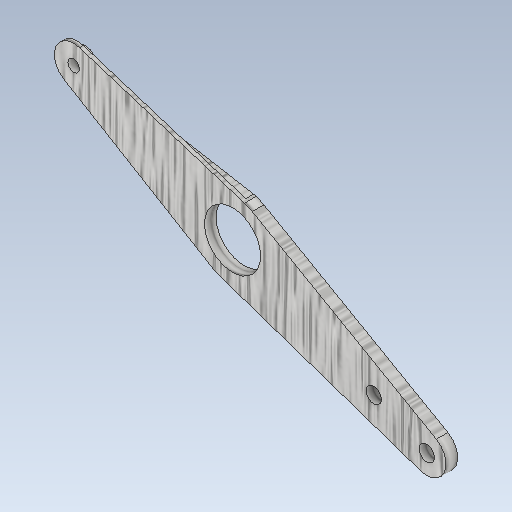
# Autodesk Inventor part: アーム中間節
Saved by Autodesk Inventor 2020 (Build 240168000, 168)
## iProperties
Created: 2019-12-03
Part Number: アーム中間節
Material: アルミニウム 7075
Document SubType Name: Modeling
Designer: tanjihayato
Density: 2.81 g/cm^3
Appearance: サテン - ブラシ仕上げ 重厚
Mass: 8.5012 g
Surface Area: 39.9096 cm^2
Volume: 3.02534 cm^3
Author: tanjihayato
Autodesk Inventor part; units mm, degrees
note: some values were not read from the file. Chosen so that the rebuilt part matches the saved one: sketch regions of "押し出し1"; sketch regions of "押し出し2".
ref_plane "YZ Plane" through (0, 0, 0) normal (1, 0, 0) x (0, 1, 0)
ref_plane "XZ Plane" through (0, 0, 0) normal (0, 1, 0) x (-1, 0, 0)
ref_plane "XY Plane" through (0, 0, 0) normal (0, 0, 1) x (1, 0, 0)
sketch "スケッチ1" plane through (0, 0, 0) normal (0, 0, 1) x (1, 0, 0)
  line L0 (-170.6512, -31.4118) -> (202.8656, -31.4118) construction
  circle A0 centre (-14, -17.4118) radius 14 construction
  circle A1 centre (14, -17.4118) radius 14 construction
  circle A2 centre (-28.0204, 0.0121) radius 20.05 construction
  circle A3 centre (-28.0204, 0.0121) radius 5.05 construction
  circle A4 centre (8.8763, 3.8907) radius 32.05 construction
  circle A5 centre (8.8763, 3.8907) radius 10.1 construction
  circle A6 centre (54.047, 13.5882) radius 36.1 construction
  line L1 (-170.915, -81.4118) -> (490.0044, -81.4118)
  circle A7 centre (-28.0204, 0.0121) radius 22.342 construction
  circle A8 centre (-39.4931, 19.1835) radius 14 construction
  circle A9 centre (-49.0547, 7.5438) radius 14 construction
  circle A10 centre (-49.0547, -7.5196) radius 14 construction
  circle A11 centre (-39.4931, -19.1593) radius 14 construction
  circle A12 centre (8.8763, 3.8907) radius 33.05 construction
  circle A13 centre (54.047, 13.5882) radius 38.1 construction
  line L2 (-11.5565, -29.1593) -> (4.2969, -29.1593) construction
  line L3 (-67.2952, 44.8622) -> (-67.2952, -57.3934) construction
  line L4 (-149.4523, -1.6098) -> (-132.6633, -31.6026)
  line L5 (-132.7701, -31.4118) -> (-132.7701, 74.0456)
  circle A14 centre (-11.4931, -19.1593) radius 14 construction
  line L6 (-197.2268, -33.1593) -> (179.6604, -33.1593) construction
  circle A15 centre (54.047, 13.5882) radius 4.025 construction
  circle A16 centre (54.047, 13.5882) radius 6 construction
  circle A17 centre (-39.4931, 19.1835) radius 5
  circle A18 centre (-49.0547, 7.5438) radius 5
  circle A19 centre (-49.0547, -7.5196) radius 5
  circle A20 centre (-39.4931, -19.1593) radius 5
  circle A21 centre (-39.4931, 19.1835) radius 8 construction
  circle A22 centre (-49.0547, 7.5438) radius 8 construction
  circle A23 centre (-49.0547, -7.5196) radius 8 construction
  circle A24 centre (-39.4931, -19.1593) radius 8 construction
  circle A25 centre (-28.0204, 0.0121) radius 4.5
  circle A26 centre (8.8763, 3.8907) radius 7.5
  line L7 (-17.5497, 32.3149) -> (-46.3578, 15.0755) construction
  line L8 (-46.3578, 15.0755) -> (-51.7515, 0.0121) construction
  line L9 (-51.7515, 0.0121) -> (-46.3578, -15.0513) construction
  line L10 (-46.3578, -15.0513) -> (-37.9391, -20.0892) construction
  circle A27 centre (-32.6283, 23.2915) radius 1.3
  circle A28 centre (-46.3578, 15.0755) radius 1.3
  circle A29 centre (-51.7515, 0.0121) radius 1.3
  circle A30 centre (-46.3578, -15.0513) radius 1.3
  circle A31 centre (-32.6283, -23.2673) radius 1.3
  line L11 (-67.2952, 23.1796) -> (-67.2952, -18.1327)
  arc A32 (79.2003, -37.212) -> (87.3507, -31.2711) centre (80.4159, -30.3183) ccw
  arc A33 (8.1864, 50.8943) -> (0.9804, 51.9708) centre (3.7003, 45.5208) ccw
  line L12 (-52.2685, -33.1593) -> (56.2168, -33.1593)
  line L13 (56.2168, -33.1593) -> (79.2003, -37.212)
  arc A34 (92.7831, 8.2659) -> (29.742, 44.2162) centre (54.047, 13.5882) ccw
  line L14 (87.3507, -31.2711) -> (92.7831, 8.2659)
  line L15 (0.9804, 51.9708) -> (-67.2952, 23.1796)
  circle A35 centre (34.0114, -24.0061) radius 4.5 construction
  circle A36 centre (34.0114, -24.0061) radius 1.5
  circle A37 centre (-21.4477, 26.0369) radius 4.5 construction
  circle A38 centre (-21.4477, 26.0369) radius 1.5
  circle A39 centre (-56.0504, 23.0377) radius 1.5
  circle A40 centre (-56.0504, 23.0377) radius 3 construction
  circle A41 centre (-56.0504, 23.0377) radius 4.5 construction
  circle A42 centre (-64.2952, 0.0121) radius 1.5
  circle A43 centre (-64.2952, 0.0121) radius 3 construction
  circle A44 centre (-64.2952, 0.0121) radius 4.3311 construction
  line L16 (54.047, 13.5882) -> (99.37, -7.5264)
  line L17 (99.37, -7.5264) -> (58.3399, 10.9541)
  line L18 (58.3399, 10.9541) -> (30.7326, 32.4678)
  line L19 (30.7326, 32.4678) -> (54.047, 13.5882)
  line L20 (99.37, -7.5264) -> (491.4359, -184.1173)
  line L21 (-183.2789, 162.2213) -> (-183.2789, -125.2315)
  line L22 (516.7211, 155.5913) -> (516.7211, -155.5644)
  circle A45 centre (99.37, -7.5264) radius 7.25
  line L23 (149.518, -30.1136) -> (397.5027, -198.9436) construction
  line L24 (220.2014, -78.2354) -> (225.3858, -8.4277) construction
  circle A46 centre (3.7003, 45.5208) radius 4
  circle A47 centre (135.8413, -23.9534) radius 2
  circle A48 centre (149.518, -30.1136) radius 2
  arc A49 (147.9092, -34.8477) -> (151.9972, -25.7715) centre (149.518, -30.1136) ccw
  line L25 (147.9092, -34.8477) -> (96.0719, -17.2312)
  line L26 (151.9972, -25.7715) -> (104.4523, 1.3749)
  circle A50 centre (30.7326, 32.4678) radius 2
  circle A51 centre (-16.1798, -24.0771) radius 4.5 construction
  circle A52 centre (-16.1798, -24.0771) radius 1.5
  line L27 (-67.2952, -18.1327) -> (-52.2685, -33.1593)
  circle A53 centre (-56.0504, -23.0135) radius 1.5
  circle A54 centre (-56.0504, -23.0135) radius 3 construction
  circle A55 centre (30.7326, 32.4678) radius 4
  arc A56 (56.8403, 15.6972) -> (51.3644, 11.3402) centre (54.047, 13.5882) ccw construction
  line L28 (96.4916, -6.1854) -> (101.9705, -5.7041) construction
  line L29 (101.9705, -5.7041) -> (99.6479, -10.6896) construction
  line L30 (99.6479, -10.6896) -> (96.4916, -6.1854) construction
  circle A57 centre (99.6479, -10.6896) radius 1.5
  circle A58 centre (101.9705, -5.7041) radius 1.5
  circle A59 centre (96.4916, -6.1854) radius 1.5
  circle A60 centre (99.37, -7.5264) radius 6
  arc A61 (97.7876, -15.8778) -> (97.5111, 0.7679) centre (99.37, -7.5264) ccw
  arc A62 (56.8403, 15.6972) -> (97.5111, 0.7679) centre (88.7632, 39.7996) ccw
  arc A63 (51.3644, 11.3402) -> (97.7876, -15.8778) centre (112.6811, 62.7237) ccw
  circle A64 centre (54.047, 13.5882) radius 8.5 construction
  line L31 (102.9595, 0.1786) -> (57.6365, 21.2931) construction
  line L32 (50.4575, 5.8833) -> (95.7806, -15.2313) construction
  circle A65 centre (12.7384, 41.2415) radius 3 construction
  circle A66 centre (12.7384, 41.2415) radius 4.5 construction
  circle A67 centre (12.7384, 41.2415) radius 1.5
  circle A68 centre (80.4159, -30.3183) radius 4
  circle A69 centre (69.7531, -26.0108) radius 1.5
  circle A70 centre (69.7531, -26.0108) radius 4.5 construction
  circle A71 centre (-56.0504, -23.0135) radius 4.5 construction
  line L33 (8.1864, 50.8943) -> (15.9809, 44.3871)
  arc A72 (15.9809, 44.3871) -> (29.742, 44.2162) centre (22.9664, 52.7545) ccw
  circle A73 centre (-5.4761, 38.5895) radius 1.5
  circle A74 centre (-5.4761, 38.5895) radius 4.5 construction
  circle A75 centre (54.047, 13.5882) radius 50 construction
  circle A76 centre (3.7003, 45.5208) radius 2
  circle A77 centre (80.4159, -30.3183) radius 2
  circle A78 centre (54.047, 13.5882) radius 1.5
  circle A79 centre (58.3399, 10.9541) radius 1.5
  circle A80 centre (58.3399, 10.9541) radius 3
  arc A81 (59.8474, 15.7214) -> (55.7687, 6.6659) centre (58.3399, 10.9541) ccw
  line L34 (94.099, -16.3172) -> (55.7687, 6.6659)
  line L35 (59.8474, 15.7214) -> (102.4604, 2.2467)
  arc A82 (104.4523, 1.3749) -> (102.4604, 2.2467) centre (99.37, -7.5264) ccw
  arc A83 (94.099, -16.3172) -> (96.0719, -17.2312) centre (99.37, -7.5264) ccw
  circle A84 centre (30.7326, 32.4678) radius 5.025
  circle A85 centre (30.7326, 32.4678) radius 8.025
  circle A86 centre (58.3399, 10.9541) radius 4.025
  circle A87 centre (58.3399, 10.9541) radius 7.025
  line L36 (25.9827, 25.9995) -> (54.1819, 5.2918)
  line L37 (53.3095, 15.8577) -> (37.1861, 27.6978)
  line L38 (65.3516, 11.3852) -> (66.2721, -3.5865)
  line L39 (66.2721, -3.5865) -> (54.1819, 5.2918)
  line L40 (66.4799, 8.6117) -> (69.0337, -1.2879)
  line L41 (66.4799, 8.6117) -> (101.8062, 2.4535)
  point P0 (0, 0)
  point P1 (0, 0)
  point P2 (-49.0547, 7.5438)
  point P3 (-49.0547, -7.5196)
  dimension "d88" = 100
  dimension "d0" = 40.1
  dimension "d1" = 10.1
  dimension "d2" = 64.1
  dimension "d3" = 20.2
  dimension "d4" = 72.2
  dimension "d5" = 95
  dimension "d6" = 44.684
  dimension "d7" = 28
  dimension "d8" = 28
  dimension "d9" = 28
  dimension "d10" = 28
  dimension "d11" = 1
  dimension "d12" = 2
  dimension "d13" = 4
  dimension "d14" = 8.05
  dimension "d15" = 12
  dimension "d16" = 10
  dimension "d17" = 10
  dimension "d18" = 10
  dimension "d19" = 10
  dimension "d20" = 3
  dimension "d21" = 3
  dimension "d22" = 3
  dimension "d23" = 3
  dimension "d24" = 9
  dimension "d25" = 15
  dimension "d26" = 2.6
  dimension "d27" = 2.6
  dimension "d28" = 2.6
  dimension "d29" = 2.6
  dimension "d30" = 2.6
  dimension "d31" = 1
  dimension "d32" = 9
  dimension "d33" = 3
  dimension "d34" = 9
  dimension "d35" = 3
  dimension "d36" = 3
  dimension "d37" = 6
  dimension "d38" = 9
  dimension "d39" = 3
  dimension "d40" = 6
  dimension "d41" = 50
  dimension "d42" = 45
  dimension "d43" = 35
  dimension "d44" = 30
  dimension "d45" = 39
  dimension "d46" = 430
  dimension "d47" = 700
  dimension "d48" = 14.5
  dimension "d49" = 300
  dimension "d50" = 10
  dimension "d51" = 70
  dimension "d52" = 120
  dimension "d53" = 140
  dimension "d54" = 8
  dimension "d55" = 4
  dimension "d56" = 4
  dimension "d57" = 15
  dimension "d58" = 40
  dimension "d59" = 10
  dimension "d60" = 4
  dimension "d61" = 9
  dimension "d62" = 3
  dimension "d63" = 3
  constraints: 84 centre point, 84 end point, 60 tangent, 47 coincident, 39 point on circle, 15 point on line, 4 midpoint, 4 vertical, 2 collinear, 2 horizontal, 1 parallel, 1 vertical alignment, 23 other
  measures "d0" diameter of A2
  measures "d1" diameter of A3
  measures "d2" diameter of A4
  measures "d3" diameter of A5
  measures "d4" diameter of A6
  measures "d5" distance from line of L1 A6.centre
  measures "d6" diameter of A7
  measures "d7" diameter of A8
  measures "d8" diameter of A9
  measures "d9" diameter of A10
  measures "d10" diameter of A11
  measures "d11" radial gap between concentric circles of A4 A12
  measures "d12" radial gap between concentric circles of A6 A13
  measures "d13" distance between parallel lines of L6 L2
  measures "d14" diameter of A15
  measures "d15" diameter of A16
  measures "d16" diameter of A17
  measures "d17" diameter of A18
  measures "d18" diameter of A19
  measures "d19" diameter of A20
  measures "d20" radial gap between concentric circles of A17 A21
  measures "d24" diameter of A25
  measures "d25" diameter of A26
  measures "d26" diameter of A27
  measures "d27" diameter of A28
  measures "d28" diameter of A29
  measures "d29" diameter of A30
  measures "d30" diameter of A31
  measures "d31" radial gap between concentric circles of A13 A34
  measures "d32" diameter of A35
  measures "d33" diameter of A36
  measures "d34" diameter of A37
  measures "d35" diameter of A38
  measures "d36" diameter of A39
  measures "d37" diameter of A40
  measures "d38" diameter of A41
  measures "d39" diameter of A42
  measures "d40" diameter of A43
  measures "d41" distance of L16.start L16.end
  measures "d42" distance of L16.end L17.end
  measures "d43" distance of L17.end L18.end
  measures "d44" distance of L18.end L16.start
  measures "d45" angle of L0 L19
  measures "d46" distance of L16.end L20.end
  measures "d47" distance between parallel lines of L22 L21
  measures "d48" diameter of A45
  measures "d49" distance of L23.start L23.end
  measures "d50" angle of L20 L23
  measures "d51" distance of L24.start L24.end
  measures "d52" angle of L23 L24
  measures "d53" distance of L16.end L24.start
  measures "d54" diameter of A46
  measures "d55" diameter of A47
  measures "d56" diameter of A48
  measures "d57" distance of L23.start A47.centre
  measures "d58" distance of A47.centre A45.centre
  measures "d59" diameter of A49
  measures "d60" diameter of A50
  measures "d61" diameter of A51
  measures "d62" diameter of A52
  measures "d63" diameter of A53
extrude "押し出し1" add sketch "スケッチ1" along normal blind 3 contours L35 L41 L14 | L14 L41 L40 L16 L38 A87 L35 | L34 L40 A62 L17 L14 | L14 L17 A45 L20 A61 A63 L34 | A63 A61 L20 A47 A48 A49 L25 A83 L34 | L41 L35 A82 L26 A49 L20 A48 A47 A61 A62 L14 | L14 A62 L16 L40 L41 | A87 L16 A62 A86 A78 A81 L35 | L17 A62 L16 L14 | L14 L16 A45 L17 | L34 L38 A62 L40 | L34 A87 A62 L38 | A62 A61 L20 A45 L16 L14 | L14 L16 A62 | L38 L16 A87 | A62 L40 L17 | L17 L40 L16 A62 | A62 L38 L17 L40 | A81 A63 | A63 A81 A78 A86 L17 A62 A87 L34 | A62 A87 L17 L38 | L40 L17 L38 L16 | A78 A86 L18 A81 | L38 L17 A87 L16 | A62 L17 A87 | A86 A62 A80 L18 A78 | A78 L18 A86 | L18 A86 L16 A81 | A87 L17 A62 L16 | A81 L16 A86 A78 | L17 A86 L16 A62 | A86 A62 A80 | L18 A78 L16 A86 | L16 A86 A62 | A86 L16 A78 | A78 L16 A80 L17 A86 | L17 A80 L16 A86 | L18 A80 L16 A78 | A80 A62 | A62 A80 L16 A79 L18 | L16 A80 A62 A86 | A80 L16 L18 A79 L17 | L17 A79 L16 A80 | L18 L16 A80 | L16 A79 L18
extrude "押し出し2" cut sketch "スケッチ1" along normal blind 2 contours L35 L41 L14 | L14 L41 L40 L16 L38 A87 L35 | A87 L16 A62 A86 A78 A81 L35 | L34 L38 A62 L40 | L34 A87 A62 L38 | L38 L16 A87 | A62 L38 L17 L40 | A81 A63 | A63 A81 A78 A86 L17 A62 A87 L34 | A62 A87 L17 L38 | L40 L17 L38 L16 | A78 A86 L18 A81 | L38 L17 A87 L16 | A62 L17 A87 | A86 A62 A80 L18 A78 | A78 L18 A86 | L18 A86 L16 A81 | A87 L17 A62 L16 | A81 L16 A86 A78 | L17 A86 L16 A62 | A86 A62 A80 | L18 A78 L16 A86 | L16 A86 A62 | A86 L16 A78 | A78 L16 A80 L17 A86 | L17 A80 L16 A86 | L18 A80 L16 A78 | L16 A80 A62 A86
sketch "スケッチ3" plane through (0, 0, 0) normal (0, 0, -1) x (-1, 0, 0)
  line L0 (-66.4799, 8.6117) -> (-101.8062, 2.4535) projected
  line L1 (-102.4604, 2.2467) -> (-101.8062, 2.4535) projected
  arc A0 (-102.4604, 2.2467) -> (-104.4523, 1.3749) centre (-99.37, -7.5264) ccw projected
  line L2 (-151.9972, -25.7715) -> (-104.4523, 1.3749) projected
  arc A1 (-151.9972, -25.7715) -> (-147.9092, -34.8477) centre (-149.518, -30.1136) ccw projected
  line L3 (-96.0719, -17.2312) -> (-147.9092, -34.8477) projected
  arc A2 (-96.0719, -17.2312) -> (-94.099, -16.3172) centre (-99.37, -7.5264) ccw projected
  line L4 (-69.0337, -1.2879) -> (-94.099, -16.3172) projected
  line L5 (-69.0337, -1.2879) -> (-66.4799, 8.6117) projected
  circle A3 centre (-135.8413, -23.9534) radius 2 projected
  circle A4 centre (-149.518, -30.1136) radius 2 projected
  circle A5 centre (-99.37, -7.5264) radius 7.25 projected
  arc A6 (-101.5559, -0.6137) -> (-102.9648, -1.2303) centre (-99.37, -7.5264) ccw
  line L6 (-101.5559, -0.6137) -> (-101.0932, -0.4674)
  line L7 (-101.0932, -0.4674) -> (-70.5466, 4.8575)
  line L8 (-70.5466, 4.8575) -> (-71.6313, 0.6525)
  line L9 (-71.6313, 0.6525) -> (-95.6417, -13.7443)
  arc A7 (-97.0372, -14.3908) -> (-95.6417, -13.7443) centre (-99.37, -7.5264) ccw
  line L10 (-97.0372, -14.3908) -> (-148.8745, -32.0072)
  arc A8 (-150.5097, -28.3767) -> (-148.8745, -32.0072) centre (-149.518, -30.1136) ccw
  line L11 (-150.5097, -28.3767) -> (-102.9648, -1.2303)
  arc A9 (-131.2941, -26.0327) -> (-134.3851, -19.1702) centre (-135.8413, -23.9534) ccw
  arc A10 (-109.2571, -4.823) -> (-103.8976, -16.7222) centre (-99.37, -7.5264) ccw
  arc A11 (-89.4275, -10.0182) -> (-93.477, 0.8602) centre (-99.37, -7.5264) ccw
  point P0 (0, 0)
  dimension "d111" = 3
  dimension "d113" = 3
  dimension "d114" = 3
  dimension "d115" = 3
  constraints: 12 end point, 12 point on circle, 6 centre point, 6 point on line, 8 other
  measures "d111" distance between parallel lines of L2 L11
  measures "d113" radial gap between concentric circles of A3 A9
  measures "d114" radial gap between concentric circles of A10 A5
  measures "d115" radial gap between concentric circles of A11 A5
extrude "押し出し3" cut sketch "スケッチ3" against normal blind 2 contours L11 A10 L10 A9 | A11 L7 L8 L9
fillet "フィレット1" radius 2 8 edges at (134.3851, -19.1702, 1) (131.2941, -26.0327, 1) (103.8976, -16.7222, 1) (109.2571, -4.823, 1) (93.477, 0.8602, 1) (89.4275, -10.0182, 1) (71.6313, 0.6525, 1) (70.5466, 4.8575, 1)
sketch "スケッチ4" plane through (0, 0, 0) normal (0, 0, -1) x (-1, 0, 0)
  arc A0 (-89.1684, -6.5314) -> (-91.0011, -1.6084) centre (-99.37, -7.5264) ccw projected
  arc A1 (-89.7115, 1.5167) -> (-91.0011, -1.6084) centre (-89.3681, -0.4536) ccw projected
  line L0 (-89.7115, 1.5167) -> (-73.6012, 4.325) projected
  arc A2 (-71.3211, 1.8552) -> (-73.6012, 4.325) centre (-73.2577, 2.3548) ccw projected
  line L1 (-71.3211, 1.8552) -> (-71.4265, 1.4465) projected
  arc A3 (-72.3346, 0.2308) -> (-71.4265, 1.4465) centre (-73.3631, 1.9461) ccw projected
  line L2 (-72.3346, 0.2308) -> (-86.1494, -8.0526) projected
  arc A4 (-89.1684, -6.5314) -> (-86.1494, -8.0526) centre (-87.1779, -6.3373) ccw projected
  arc A5 (-130.8782, -23.3469) -> (-132.0981, -20.6385) centre (-135.8413, -23.9534) ccw projected
  arc A6 (-131.5925, -17.5757) -> (-132.0981, -20.6385) centre (-130.6008, -19.3125) ccw projected
  line L3 (-131.5925, -17.5757) -> (-112.5765, -6.7182) projected
  arc A7 (-109.5905, -8.3034) -> (-112.5765, -6.7182) centre (-111.5848, -8.4551) ccw projected
  arc A8 (-109.5905, -8.3034) -> (-106.725, -14.6655) centre (-99.37, -7.5264) ccw projected
  arc A9 (-107.5166, -17.9521) -> (-106.725, -14.6655) centre (-108.1601, -16.0585) ccw projected
  line L4 (-107.5166, -17.9521) -> (-128.2494, -24.998) projected
  arc A10 (-130.8782, -23.3469) -> (-128.2494, -24.998) centre (-128.893, -23.1043) ccw projected
  line L5 (-66.4799, 8.6117) -> (-101.8062, 2.4535) projected
  line L6 (-102.4604, 2.2467) -> (-101.8062, 2.4535) projected
  arc A11 (-102.4604, 2.2467) -> (-104.4523, 1.3749) centre (-99.37, -7.5264) ccw projected
  line L7 (-151.9972, -25.7715) -> (-104.4523, 1.3749) projected
  arc A12 (-151.9972, -25.7715) -> (-147.9092, -34.8477) centre (-149.518, -30.1136) ccw projected
  line L8 (-96.0719, -17.2312) -> (-147.9092, -34.8477) projected
  arc A13 (-96.0719, -17.2312) -> (-94.099, -16.3172) centre (-99.37, -7.5264) ccw projected
  line L9 (-69.0337, -1.2879) -> (-94.099, -16.3172) projected
  line L10 (-69.0337, -1.2879) -> (-66.4799, 8.6117) projected
  circle A14 centre (-135.8413, -23.9534) radius 2 projected
  circle A15 centre (-149.518, -30.1136) radius 2 projected
  circle A16 centre (-99.37, -7.5264) radius 7.25 projected
  arc A17 (-55.7687, 6.6659) -> (-59.8474, 15.7214) centre (-58.3399, 10.9541) ccw projected
  line L11 (-101.8062, 2.4535) -> (-59.8474, 15.7214) projected
  line L12 (-66.4799, 8.6117) -> (-101.8062, 2.4535) projected
  line L13 (-69.0337, -1.2879) -> (-66.4799, 8.6117) projected
  line L14 (-55.7687, 6.6659) -> (-69.0337, -1.2879) projected
  circle A18 centre (-58.3399, 10.9541) radius 3 projected
  arc A19 (-151.9972, -25.7715) -> (-147.9092, -34.8477) centre (-149.518, -30.1136) ccw projected
  line L15 (-151.9972, -25.7715) -> (-104.4523, 1.3749) projected
  arc A20 (-102.4604, 2.2467) -> (-104.4523, 1.3749) centre (-99.37, -7.5264) ccw projected
  line L16 (-102.4604, 2.2467) -> (-59.8474, 15.7214) projected
  arc A21 (-55.7687, 6.6659) -> (-59.8474, 15.7214) centre (-58.3399, 10.9541) ccw projected
  line L17 (-55.7687, 6.6659) -> (-94.099, -16.3172) projected
  arc A22 (-96.0719, -17.2312) -> (-94.099, -16.3172) centre (-99.37, -7.5264) ccw projected
  line L18 (-96.0719, -17.2312) -> (-147.9092, -34.8477) projected
  circle A23 centre (-135.8413, -23.9534) radius 2 projected
  circle A24 centre (-149.518, -30.1136) radius 2 projected
  circle A25 centre (-99.37, -7.5264) radius 7.25 projected
  circle A26 centre (-58.3399, 10.9541) radius 1.5 projected
  arc A27 (-102.2781, 4.4966) -> (-101.8062, 2.4535) centre (-101.9865, 3.4879) ccw
  arc A28 (-69.0337, -1.2879) -> (-67.4295, -2.4205) centre (-68.017, -1.5502) ccw
  line L19 (-66.4799, 8.6117) -> (-101.8062, 2.4535) projected
  line L20 (-102.2781, 4.4966) -> (-60.0063, 16.718)
  line L21 (-67.4295, -2.4205) -> (-54.983, 5.981)
  arc A29 (-54.983, 5.981) -> (-60.0063, 16.718) centre (-58.3399, 10.9541) ccw
  point P0 (0, 0)
  dimension "d119" = 2.1
  dimension "d120" = 2.1
  dimension "d121" = 1
  constraints: 8 point on circle, 6 tangent, 4 end point, 3 centre point, 2 point on line, 1 coincident
  measures "d119" diameter of A27
  measures "d120" diameter of A28
  measures "d121" radial gap between concentric circles of A29 A17
